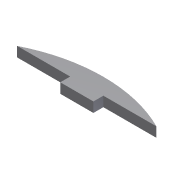
# Autodesk Inventor part: OpenROV_Dev_EChassis_Blinder
Saved by Autodesk Inventor 2012 (Build 160160000, 160)
## iProperties
Created: 2012-08-11
Part Number: OpenROV_Dev_EChassis_Blinder
Material: Default
Document SubType Name: Modeling
Designer: user
Density: 1 g/cm^3
Author: user
Autodesk Inventor part; units mm, degrees
ref_plane "YZ Plane" through (0, 0, 0) normal (1, 0, 0) x (0, 1, 0)
ref_plane "XZ Plane" through (0, 0, 0) normal (0, 1, 0) x (-1, 0, 0)
ref_plane "XY Plane" through (0, 0, 0) normal (0, 0, 1) x (1, 0, 0)
sketch "Sketch1" plane through (0, 0, 0) normal (0, 0, 1) x (1, 0, 0)
  arc A0 (21, 42.0476) -> (-21, 42.0476) centre (0, 0) ccw
  line L0 (-5, 42.0476) -> (-5, 39.0476)
  line L1 (-5, 39.0476) -> (5, 39.0476)
  line L2 (5, 39.0476) -> (5, 42.0476)
  line L3 (-21, 42.0476) -> (-5, 42.0476)
  line L4 (5, 42.0476) -> (21, 42.0476)
  dimension "d0" = 94
  dimension "d2" = 3
  dimension "d3" = 10
  dimension "d4" = 5
  dimension "d8" = 16
  dimension "d9" = 16
  constraints: 10 end point, 3 perpendicular, 2 horizontal, 2 point on circle, 1 centre point, 1 coincident, 1 parallel
  measures "d0" diameter of A0
  measures "d2" distance between parallel lines of L1 L3
  measures "d3" distance between parallel lines of L2 L0
  measures "d4" distance from line of point (0, 0) L0
  measures "d8" distance of L3.start L0.start
  measures "d9" distance of L2.end L4.end
extrude "Extrusion1" add sketch "Sketch1" along normal blind 3
body "Solid1"
